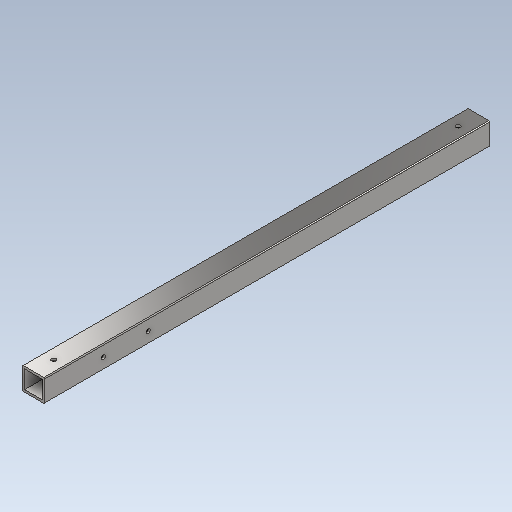
# Autodesk Inventor part: support_frame_x
Saved by Autodesk Inventor 2021 (Build 250183000, 183)
## iProperties
Created: 2021-05-24
Part Number: support_frame_x
Material: Steel, Mild
Document SubType Name: Modeling
Designer: Watchdog
Density: 7.85 g/cm^3
Appearance: Semi-Polished
Mass: 6667.65 g
Surface Area: 3405.31 cm^2
Volume: 849.382 cm^3
Author: Watchdog
Autodesk Inventor part; units mm, degrees
ref_plane "YZ Plane" through (0, 0, 0) normal (1, 0, 0) x (0, 1, 0)
ref_plane "XZ Plane" through (0, 0, 0) normal (0, 1, 0) x (-1, 0, 0)
ref_plane "XY Plane" through (0, 0, 0) normal (0, 0, 1) x (1, 0, 0)
sketch "Sketch1" plane through (0, 0, 0) normal (0, 0, 1) x (1, 0, 0)
  line L0 (-25, 25) -> (25, 25)
  line L1 (25, 25) -> (25, -25)
  line L2 (25, -25) -> (-25, -25)
  line L3 (-25, -25) -> (-25, 25)
  line L4 (20, 20) -> (-20, 20)
  line L5 (-20, 20) -> (-20, -20)
  line L6 (-20, -20) -> (20, -20)
  line L7 (20, -20) -> (20, 20)
  point P0 (0, 0)
  dimension "d0" = 50
  dimension "d1" = 50
  dimension "d2" = 25
  dimension "d3" = 25
  dimension "d4" = 5
  constraints: 16 end point, 4 parallel, 2 perpendicular, 1 horizontal, 3 other
  measures "d0" distance of L0.start L0.end
  measures "d1" distance of L2.end L0.start
  measures "d2" distance from line of L0 point (0, 0)
  measures "d3" distance from line of point (0, 0) L3
  measures "d4" distance between parallel lines of L0 L4
extrude "Extrusion1" add sketch "Sketch1" along normal blind 990
fillet "Fillet1" radius 2 4 edges at (25, 25, 495) (-25, 25, 495) (25, -25, 495) (-25, -25, 495)
sketch "Sketch2" plane through (-23, 25, 0) normal (0, 1, 0) x (1, 0, 0)
  line L0 (46, 0) -> (0, 0) projected
  line L1 (46, -990) -> (0, -990) projected
  point P0 (23, 0)
  point P1 (23, -45)
  point P2 (23, -945)
  dimension "d8" = 45
  dimension "d9" = 0
  dimension "d10" = 45
  dimension "d11" = 0
  measures "d8" distance from line of point (23, -45) L0
  measures "d9" horizontal distance of point (23, -45) point (23, 0)
  measures "d10" distance from line of L1 point (23, -945)
  measures "d11" horizontal distance of point (23, -945) point (23, 0)
hole "endHoles" at (0, 25, 45) at (0, 25, 945) direction (0, -1, 0) diameter 10 depth 5
sketch "Sketch3" plane through (25, -23, 0) normal (1, 0, 0) x (0, 0, -1)
  point P0 (0, 23)
  point P1 (-860, 23)
  point P2 (-760, 23)
  dimension "d19" = 860
  dimension "d20" = 760
  dimension "d21" = 0
  dimension "d22" = 0
  measures "d19" distance of point (0, 23) point (-860, 23)
  measures "d20" distance of point (0, 23) point (-760, 23)
  measures "d21" vertical distance of point (0, 23) point (-760, 23)
  measures "d22" vertical distance of point (0, 23) point (-860, 23)
hole "clampHoles" at (25, 0, 860) at (25, 0, 760) direction (-1, 0, 0) diameter 10 end through all
equation "\"d0\" = w"
equation "\"d1\" = w"
equation "\"d2\" = 0.5 * d1"
equation "\"d3\" = 0.5 * d0"
equation "\"d4\" = t"
equation "\"d5\" = L + 2 * buffer"
equation "\"d7\" = fillet"
equation "\"d8\" = buffer"
equation "\"d10\" = buffer"
equation "\"d23\" = support_frame_clampHoleDiameter"
equation "\"w\" = support_frame_squareBarDimension"
equation "\"t\" = support_frame_squareBarThickness"
equation "\"fillet\" = support_frame_squareBarFillet"
equation "\"support_frame_endHoleBuffer\" = 45"
equation "\"buffer\" = support_frame_endHoleBuffer"
equation "\"hoop_angle_z\" = 45deg"
equation "\"hoop_bearing_length\" = 5deg"
equation "\"hoop_cable_diam\" = 5"
equation "\"hoop_cable_pulley_diam\" = 22"
equation "\"hoop_thickness_large\" = 4"
equation "\"hoop_thickness_medium\" = 3.2"
equation "\"hoop_thickness_small\" = 2"
equation "\"hoop_width_large\" = 51"
equation "\"hoop_width_medium\" = 33.7"
equation "\"hoop_width_small\" = 25.4"
equation "\"rack_tooth_addendum\" = 5"
equation "\"rack_tooth_dedendum\" = 5"
equation "\"rack_tooth_thickness\" = 5"
equation "\"secure_arm_angle\" = 35deg"
equation "\"secure_arm_radii\" = 9"
equation "\"support_baseClamp_platformLengthBuffer\" = 35"
equation "\"support_baseClamp_platformThickness\" = 15"
equation "\"support_baseClamp_platformWidthBuffer\" = 0"
equation "\"support_baseClamp_sleeveHoleDiameter\" = 12"
equation "\"support_baseClamp_sleeveSweepTerminationAngle\" = 55deg"
equation "\"support_baseClamp_thickness\" = 8"
equation "\"support_frame_clampHoleDiameter\" = 10"
equation "\"support_frame_squareBarFillet\" = 2"
equation "\"support_frame_squareBarThickness\" = 5"
equation "\"hoop_tabs_thickness\" = 6"
equation "\"wheelchair_deployed_length\" = 1067"
equation "\"wheelchair_deployed_height\" = 914"
equation "\"hoop_tabs_hole\" = 12"
equation "\"wheelchair_deployed_width\" = 635"
equation "\"sm_varx_pinPlate_thickness\" = 5"
equation "\"sm_varx_member_tolerance\" = 0.5"
equation "\"sm_varx_pinPlate_holeDiameter\" = 5"
equation "\"sm_varx_squareBarThickness\" = 2.5"
equation "\"hoop_bushing23_radialInterference\" = 0"
equation "\"hoop_bushing12_radialInterference\" = 0"
equation "\"hoop_bushing12_od\" = -2 * hoop_thickness_large + hoop_width_large + hoop_bushing12_radialInterference"
equation "\"wheelchatir_pos_deploy_angle_0\" = 65deg"
equation "\"wheelchatir_pos_store_angle_0\" = 90deg"
equation "\"wheelchatir_pos_deploy_angle_1\" = 20deg"
equation "\"wheelchatir_pos_store_angle_1\" = 20deg"
equation "\"hoop_bushing23_od\" = -2 * hoop_thickness_medium + hoop_width_medium + hoop_bushing23_radialInterference"
equation "\"hoop_bushing12_thickness\" = -hoop_width_medium + hoop_bushing12_od - 2 * hoop_bushing12_radialInterference"
equation "\"hoop_bushing23_thickness\" = -hoop_width_small + hoop_bushing23_od - 2 * hoop_bushing23_radialInterference"
equation "\"L\" = 900"
equation "\"support_frame_squareBarDimension\" = 50"
body "Solid1"
